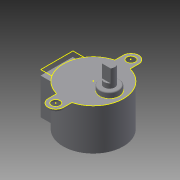
# Autodesk Inventor part: stepper motor-cheapo geared
Saved by Autodesk Inventor 2015 SP2 (Build 190223200, 223)
## iProperties
Created: 2015-05-24
Part Number: stepper motor-cheapo geared
Material: Generic
Document SubType Name: Modeling
Designer: caleb
Density: 1 g/cm^3
Appearance: Default
Author: caleb
Autodesk Inventor part; units mm, degrees
ref_plane "XZ Plane" through (0, 0, 0) normal (0, 1, 0) x (-1, 0, 0)
ref_plane "XY Plane" through (0, 0, 0) normal (0, 0, 1) x (1, 0, 0)
sketch "Sketch1" plane through (0, 0, 0) normal (0, 0, 1) x (1, 0, 0)
  circle A0 centre (0, 0) radius 2.5
  dimension "d0" = 5
  constraints: 1 centre point, 1 coincident
  measures "d0" diameter of A0
extrude "Extrusion1" add sketch "Sketch1" along normal blind 8.17
sketch "Sketch2" plane through (0, 0, 8.17) normal (0, 0, 1) x (1, 0, 0)
  circle A0 centre (0, 0) radius 2.5 construction
  circle A1 centre (0, 0) radius 2.5 construction
  line L0 (-2, -1.5) -> (2, -1.5)
  line L1 (2, -1.5) -> (2, 1.5)
  line L2 (2, 1.5) -> (-2, 1.5)
  line L3 (-2, 1.5) -> (-2, -1.5)
  line L4 (-2, -1.5) -> (2, 1.5) construction
  line L5 (2, -1.5) -> (-2, 1.5) construction
  arc A2 (-2, 1.5) -> (-2, -1.5) centre (0, 0) ccw
  arc A3 (2, 1.5) -> (-2, 1.5) centre (0, 0) ccw
  arc A4 (-2, -1.5) -> (2, -1.5) centre (0, 0) ccw
  arc A5 (2, -1.5) -> (2, 1.5) centre (0, 0) ccw
  dimension "d3" = 3
  constraints: 12 end point, 8 point on circle, 4 centre point, 2 midpoint, 2 parallel, 1 coincident, 1 horizontal, 1 perpendicular, 4 other
  measures "d3" distance of L0.end L1.end
extrude "Extrusion2" cut sketch "Sketch2" against normal blind 6 contours L0 A4 | A3 L2
sketch "Sketch3" plane through (0, 0, 0) normal (0, 0, -1) x (-1, 0, 0)
  circle A0 centre (0, 0) radius 2.5 projected
  circle A1 centre (0, 0) radius 4.55
  dimension "d6" = 9.1
  constraints: 1 centre point, 1 coincident
  measures "d6" diameter of A1
extrude "Extrusion3" add sketch "Sketch3" along normal blind 2.5 contours A0 | A1
sketch "Sketch4" plane through (0, 0, -2.5) normal (0, 0, -1) x (-1, 0, 0)
  circle A0 centre (7.55, 0) radius 14
  circle A1 centre (0, 0) radius 4.55 projected
  line L0 (4.55, 0) -> (-6.45, 0) construction
  dimension "d9" = 28
  dimension "d10" = 11
  constraints: 4 horizontal alignment, 2 end point, 1 horizontal, 3 other
  measures "d10" distance of L0.start L0.end
extrude "Extrusion4" add sketch "Sketch4" along normal blind 19.3 contours A0 | A1
fillet "Fillet1" radius 0.5 1 edges at (4.55, 0, 0)
sketch "Sketch5" plane through (-7.55, 0, -21.8) normal (0, 0, -1) x (-1, 0, 0)
  circle A0 centre (0, 0) radius 14 construction
  line L0 (11.8216, -7.5) -> (17, -7.5)
  line L1 (17, -7.5) -> (17, 7.5)
  line L2 (17, 7.5) -> (11.8216, 7.5)
  line L3 (11.8216, 7.5) -> (11.8216, -7.5)
  line L4 (11.8216, -7.5) -> (17, 7.5) construction
  line L5 (17, -7.5) -> (11.8216, 7.5) construction
  circle A1 centre (0, 0) radius 14 construction
  line L6 (17, 0) -> (-14, 0) construction
  circle A2 centre (0, 0) radius 14 construction
  point P0 (-7.55, 0)
  point P1 (14.4108, 0)
  dimension "d14" = 15
  dimension "d15" = 31
  constraints: 14 end point, 3 midpoint, 3 point on circle, 2 horizontal alignment, 2 parallel, 1 horizontal, 1 perpendicular, 1 other
  measures "d14" distance of L0.end L1.end
  measures "d15" distance of L6.start L6.end
extrude "Extrusion5" add sketch "Sketch5" against normal blind 16.8
sketch "Sketch6" plane through (-7.55, 0, -2.5) normal (0, 0, 1) x (1, 0, 0)
  circle A0 centre (0, 0) radius 14 projected
  circle A1 centre (7.55, 0) radius 4.55 construction
  arc A2 (-11.8216, -7.5) -> (-11.8216, 7.5) centre (0, 0) ccw projected
  line L0 (3.55, 13.5424) -> (3.55, 17.5)
  arc A3 (3.55, 17.5) -> (-3.55, 17.5) centre (0, 17.5) ccw
  line L1 (-3.55, 17.5) -> (-3.55, 13.5424)
  circle A4 centre (0, 17.5) radius 2
  dimension "d18" = 4
  dimension "d19" = 7.1
  dimension "d20" = 17.5
  constraints: 6 point on circle, 4 end point, 2 centre point, 2 tangent, 1 coincident, 1 parallel, 1 vertical, 1 vertical alignment
  measures "d18" diameter of A4
  measures "d19" distance between parallel lines of L0 L1
  measures "d20" distance of A0.centre A3.centre
extrude "Extrusion6" add sketch "Sketch6" against normal blind 0.86 contours A0 L1 A3 L0
mirror "Mirror1" about plane through (0, 0, 0) normal (0, 1, 0) of "Extrusion6"
sketch "Sketch7" plane through (0, 0, -2.5) normal (0, 0, 1) x (1, 0, 0)
  arc A0 (-4, -13.5424) -> (-4, 13.5424) centre (-7.55, 0) ccw projected
  point P0 (0, 0)
ref_plane "align plane" through (-7.55, 0, -2.5) normal (1, 0, 0) x (0, 1, 0)
sketch "motor front face" plane through (0, 0, -2.5) normal (0, 0, 1) x (1, 0, 0)
  circle A0 centre (-7.55, -17.5) radius 2 projected
  circle A1 centre (-7.55, 17.5) radius 2 projected
  arc A2 (-11.1, 13.5424) -> (-11.1, -13.5424) centre (-7.55, 0) ccw projected
  line L0 (-11.1, -17.5) -> (-11.1, -13.5424) projected
  arc A3 (-11.1, -17.5) -> (-4, -17.5) centre (-7.55, -17.5) ccw projected
  line L1 (-4, -13.5424) -> (-4, -17.5) projected
  arc A4 (-4, -13.5424) -> (-4, 13.5424) centre (-7.55, 0) ccw projected
  line L2 (-4, 13.5424) -> (-4, 17.5) projected
  arc A5 (-4, 17.5) -> (-11.1, 17.5) centre (-7.55, 17.5) ccw projected
  line L3 (-11.1, 17.5) -> (-11.1, 13.5424) projected
  circle A6 centre (0, 0) radius 4.55 projected
  arc A7 (-19.3716, 7.5) -> (-19.3716, -7.5) centre (-7.55, 0) ccw projected
  line L4 (-19.3716, 7.5) -> (-24.55, 7.5) projected
  line L5 (-24.55, 7.5) -> (-24.55, -7.5) projected
  line L6 (-24.55, -7.5) -> (-19.3716, -7.5) projected
body "Solid1"
